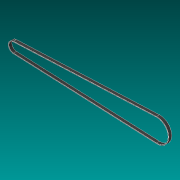
# Autodesk Inventor part: Tandriem20naar60T-696mm
Saved by Autodesk Inventor 2020.2 (Build 242310000, 310)
## iProperties
Created: 2020-05-20
Part Number: Tandriem20naar60T-696mm
Material: Rubber
Document SubType Name: Modeling
Designer: Svend
Density: 0.93 g/cm^3
Appearance: Rubber - Black
Author: Svend
Autodesk Inventor part; units mm, degrees
ref_plane "YZ Plane" through (0, 0, 0) normal (1, 0, 0) x (0, 1, 0)
ref_plane "XZ Plane" through (0, 0, 0) normal (0, 1, 0) x (-1, 0, 0)
ref_plane "XY Plane" through (0, 0, 0) normal (0, 0, 1) x (1, 0, 0)
sketch "Sketch1" plane through (0, 0, 0) normal (0, 0, 1) x (1, 0, 0)
  arc A0 (-0.3997, 8.9911) -> (-0.3997, -8.9911) centre (0, 0) ccw
  arc A1 (269.2639, -20.9793) -> (269.2639, 20.9793) centre (270.1966, 0) ccw
  line L0 (269.2639, 20.9793) -> (-0.3997, 8.9911)
  line L1 (-0.3997, -8.9911) -> (269.2639, -20.9793)
  line L2 (-0.4574, 10.2898) -> (269.2062, 22.278)
  arc A2 (269.2062, -22.278) -> (269.2062, 22.278) centre (270.1966, 0) ccw
  line L3 (269.2062, -22.278) -> (-0.4574, -10.2898)
  arc A3 (-0.4574, 10.2898) -> (-0.4574, -10.2898) centre (0, 0) ccw
  dimension "d0" = 18
  dimension "d1" = 42
  dimension "d2" = 269.93
  dimension "d3" = 1.3
  constraints: 8 end point, 8 point on circle, 4 centre point, 4 tangent, 1 coincident, 1 horizontal alignment, 3 other
  measures "d0" diameter of A0
  measures "d1" diameter of A1
  measures "d2" distance of L0.start L0.end
  measures "d3" distance between parallel lines of L0 L2
extrude "Extrusion1" add sketch "Sketch1" along normal mid plane 6
chamfer "Chamfer1" distance 0.2 angle 45 16 edges at (291.1966, 0, 3) (134.4321, -14.9852, 3) (-9, 0, 3) (134.4321, 14.9852, 3) (291.1966, 0, -3) (134.4321, 14.9852, -3) (-9, 0, -3) (134.4321, -14.9852, -3) (292.4966, 0, 3) (134.3744, 16.2839, 3) (-10.3, 0, 3) (134.3744, -16.2839, 3) (292.4966, 0, -3) (134.3744, -16.2839, -3) (-10.3, 0, -3) (134.3744, 16.2839, -3)
body "Solid1"
